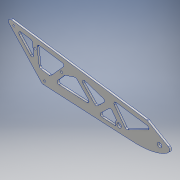
# Autodesk Inventor part: bracket1
Saved by Autodesk Inventor 2018.2 (Build 222227000, 227)
## iProperties
Created: 2018-03-05
Part Number: bracket1
Material: アルミニウム 6061
Document SubType Name: Modeling
Designer: ku_sk
Density: 2.7 g/cm^3
Appearance: アルミニウム - フラット
Mass: 423.846 g
Surface Area: 682.947 cm^2
Volume: 156.98 cm^3
Author: ku_sk
Autodesk Inventor part; units mm, degrees
ref_plane "YZ Plane" through (0, 0, 0) normal (1, 0, 0) x (0, 1, 0)
ref_plane "XZ Plane" through (0, 0, 0) normal (0, 1, 0) x (-1, 0, 0)
ref_plane "XY Plane" through (0, 0, 0) normal (0, 0, 1) x (1, 0, 0)
sketch "スケッチ2" plane through (0, 0, 0) normal (0, 1, 0) x (-1, 0, 0)
  arc A0 (320.7468, 34.8983) -> (392.1215, 71.6787) centre (243.1623, 273.099) ccw projected
  arc A1 (310.5095, 31.8959) -> (320.7468, 34.8983) centre (264.9264, 206.2785) ccw projected
  arc A2 (290.9118, 29.5172) -> (310.5095, 31.8959) centre (291.9468, 102.9093) ccw projected
  arc A3 (278.6891, 31.4878) -> (290.9118, 29.5172) centre (291.5128, 72.1352) ccw projected
  arc A4 (274.9831, 33.389) -> (278.6891, 31.4878) centre (282.4278, 43.3382) ccw projected
  arc A5 (275.4733, 39.2078) -> (274.9831, 33.389) centre (277.0456, 36.1453) ccw projected
  arc A6 (283.1253, 42.3274) -> (275.4733, 39.2078) centre (297.1464, -3.0086) ccw projected
  arc A7 (310.1184, 49.282) -> (283.1253, 42.3274) centre (369.3413, -236.446) ccw projected
  arc A8 (310.1184, 49.282) -> (326.9533, 52.7997) centre (-771.7798, 5269.0252) ccw projected
  arc A9 (326.9533, 52.7997) -> (357.98, 60.8795) centre (256.8539, 385.5961) ccw projected
  arc A10 (357.98, 60.8795) -> (391.1188, 73.3957) centre (268.9975, 346.6028) ccw projected
  arc A11 (392.1215, 71.6787) -> (391.1188, 73.3957) centre (391.5269, 72.4828) ccw projected
  circle A12 centre (287.1934, 37.1564) radius 3 projected
  circle A13 centre (359.7933, 56.2153) radius 3 projected
  arc A14 (100.5026, -29.4375) -> (303.8176, 17.6729) centre (68.6386, 570.3585) ccw projected
  arc A15 (74.9408, -30.0377) -> (100.5026, -29.4375) centre (77.5861, 401.9345) ccw projected
  arc A16 (28.1912, -23.4013) -> (74.9408, -30.0377) centre (76.0159, 145.5175) ccw projected
  arc A17 (1.2395, -11.312) -> (28.1912, -23.4013) centre (55.8939, 74.446) ccw projected
  arc A18 (-6.0217, -4.7376) -> (1.2395, -11.312) centre (16.9451, 13.3315) ccw projected
  arc A19 (-1.6159, 7.4897) -> (-6.0217, -4.7376) centre (0, 0) ccw projected
  arc A20 (17.9572, 9.9554) -> (-1.6159, 7.4897) centre (22.277, -103.2534) ccw projected
  arc A21 (84.7958, 9.311) -> (17.9572, 9.9554) centre (44.6377, -689.2581) ccw projected
  arc A22 (84.7958, 9.311) -> (126.0099, 7.0084) centre (819.0754, 12782.4716) ccw projected
  arc A23 (126.0099, 7.0084) -> (203.0122, 6.466) centre (170.258, 822.6468) ccw projected
  arc A24 (203.0122, 6.466) -> (303.8176, 17.6729) centre (174.1884, 724.7085) ccw projected
  circle A25 centre (20.0666, -1.5588) radius 5 projected
  circle A26 centre (130.4331, -10.1322) radius 5 projected
  line L0 (100.5026, -29.4375) -> (340.2835, -16.6992)
  line L1 (-3.831, 6.6355) -> (54.1787, 40.1274)
  line L2 (1137.2465, 0) -> (-1089.9509, 0) projected
  line L3 (54.1787, 40.1274) -> (443.8225, 95.0028)
  line L4 (340.2835, -16.6992) -> (443.8225, 95.0028)
  point P0 (0, 0)
  point P1 (371.2778, 57.8193)
  dimension "d7" = 30
  constraints: 8 end point, 2 point on circle, 2 tangent
  measures "d7" angle of L2 L1
extrude "押し出し3" add sketch "スケッチ2" along normal blind 5 contours A1 A2 A3 A4 A5 A6 A7 A8 A9 A10 A11 A0 | A15 A16 A17 A18 A19 L2 A25 A14 | A14 L2 L4 L0 | L2 A25 A19 A20 A21 A22 A23 A24 A14 | A14 A24 A23 A22 A21 A20 A19 L1 L3 L4 L2
fillet "フィレット2" radius 6 2 edges at (-54.1787, 2.5, 40.1274) (-340.2835, 2.5, -16.6992)
fillet "フィレット2" radius 7 1 edges at (-443.8225, 2.5, 95.0028)
sketch "スケッチ4" plane through (0, 5, 0) normal (0, 1, 0) x (1, 0, 0)
  circle A0 centre (-333.5539, 7.0426) radius 2.5
  line L0 (-53.1694, -39.5447) -> (3.831, -6.6355) projected
  line L1 (-443.8225, -95.0028) -> (-55.3327, -40.2899) projected
  line L2 (-100.5026, 29.4375) -> (-337.8548, 16.8282) projected
  line L3 (-341.9369, 14.9154) -> (-443.8225, -95.0028) projected
  circle A1 centre (-417.3739, -81.1793) radius 2.5
  point P0 (0, 0)
  dimension "d21" = 5
  dimension "d22" = 10
  dimension "d23" = 11.5
  dimension "d77" = 10
  dimension "d78" = 10
  dimension "d79" = 5
  constraints: 2 centre point
  measures "d21" diameter of A0
  measures "d22" distance from line of L2 A0.centre
  measures "d23" distance from line of L3 A0.centre
  measures "d77" distance from line of A1.centre L1
  measures "d78" distance from line of L3 A1.centre
  measures "d79" diameter of A1
sketch "スケッチ6" plane through (0, 0, 0) normal (0, -1, 0) x (1, 0, 0)
  circle A0 centre (-20.0666, -1.5588) radius 6
  circle A1 centre (-20.0666, -1.5588) radius 5 projected
  circle A2 centre (-130.4331, -10.1322) radius 6
  circle A3 centre (-130.4331, -10.1322) radius 5 projected
  point P0 (0, 0)
  dimension "d29" = 12
  dimension "d30" = 12
  constraints: 2 centre point, 2 concentric
  measures "d29" diameter of A0
  measures "d30" diameter of A2
extrude "押し出し7" cut sketch "スケッチ6" against normal through all
extrude "押し出し9" cut sketch "スケッチ4" against normal through all
sketch "スケッチ7" plane through (0, 0, 0) normal (0, -1, 0) x (1, 0, 0)
  line L0 (-412.0842, 78.4146) -> (-367.524, 72.1389)
  line L1 (-367.524, 72.1389) -> (-360.7767, 23.062)
  line L2 (-360.7767, 23.062) -> (-412.0842, 78.4146)
  line L3 (-424.3323, 92.2579) -> (-55.3327, 40.2899) projected
  line L4 (-341.9369, -14.9154) -> (-430.4423, 80.5677) projected
  line L5 (-355.1719, 70.3993) -> (-347.8097, 16.8493)
  line L6 (-347.8097, 16.8493) -> (-317.9372, 12.6422)
  line L7 (-317.9372, 12.6422) -> (-275.9537, 59.2426)
  line L8 (-275.9537, 59.2426) -> (-355.1719, 70.3993)
  line L9 (-304.865, 4.742) -> (-205.0058, -0.563)
  line L10 (-205.0058, -0.563) -> (-248.1507, 44.1788)
  line L11 (-248.1507, 44.1788) -> (-278.0912, 34.4601)
  line L12 (-278.0912, 34.4601) -> (-304.865, 4.742)
  line L13 (-100.5026, -29.4375) -> (-337.8548, -16.8282) projected
  line L14 (-193.1155, 2.9534) -> (-242.9077, 54.5886)
  line L15 (-242.9077, 54.5886) -> (-165.6606, 29.4284)
  line L16 (-165.6606, 29.4284) -> (-193.1155, 2.9534)
  line L17 (-150.8906, 41.6294) -> (-111.4803, -10.7012)
  line L18 (-111.4803, -10.7012) -> (-37.0144, 25.5916)
  line L19 (-37.0144, 25.5916) -> (-150.8906, 41.6294)
  line L20 (-153.5684, 20.2509) -> (-188.5225, -13.4556)
  line L21 (-188.5225, -13.4556) -> (-125.6693, -16.7947)
  line L22 (-125.6693, -16.7947) -> (-153.5684, 20.2509)
  point P0 (0, 0)
  dimension "d82" = 12
  dimension "d83" = 12
  dimension "d84" = 35
  dimension "d85" = 12
  dimension "d86" = 45
  dimension "d87" = 56
  dimension "d88" = 52
  dimension "d89" = 80
  dimension "d90" = 15
  dimension "d91" = 30
  dimension "d92" = 40
  dimension "d93" = 100
  dimension "d94" = 43
  dimension "d95" = 6
  dimension "d96" = 28
  dimension "d97" = 11
  dimension "d99" = 90
  dimension "d100" = 12
  dimension "d101" = 45
  dimension "d102" = 34
  dimension "d103" = 115
  dimension "d104" = 45
  dimension "d108" = 12
  dimension "d109" = 15
  dimension "d110" = 15
  constraints: 40 end point, 11 parallel, 2 point on line, 1 collinear
  measures "d82" distance between parallel lines of L0 L3
  measures "d83" distance between parallel lines of L4 L2
  measures "d84" angle of L2 L1
  measures "d85" distance between parallel lines of L5 L1
  measures "d86" distance of L0.start L0.end
  measures "d87" angle of L7 L8
  measures "d88" distance between parallel lines of L8 L6
  measures "d89" distance of L7.end L5.start
  measures "d90" distance between parallel lines of L12 L7
  measures "d91" angle of L12 L11
  measures "d92" distance of L11.end L9.start
  measures "d93" distance of L9.start L9.end
  measures "d94" angle of L9 L10
  measures "d95" distance from line of L9.start L6
  measures "d96" angle of L14 L15
  measures "d97" distance between parallel lines of L10 L14
  measures "d99" angle of L14 L16
  measures "d100" distance between parallel lines of L19 L3
  measures "d101" angle of L17 L19
  measures "d102" angle of L18 L19
  measures "d103" distance of L18.end L17.start
  measures "d104" distance of point (0, 0) L18.end
  measures "d108" distance between parallel lines of L9 L21
  measures "d109" distance between parallel lines of L17 L22
  measures "d110" distance between parallel lines of L16 L20
extrude "押し出し10" cut sketch "スケッチ7" against normal through all
fillet "フィレット3" radius 5 20 edges at (-412.0842, 2.5, 78.4146) (-355.1719, 2.5, 70.3993) (-278.0912, 2.5, 34.4601) (-242.9077, 2.5, 54.5886) (-150.8906, 2.5, 41.6294) (-111.4803, 2.5, -10.7012) (-193.1155, 2.5, 2.9534) (-317.9372, 2.5, 12.6422) (-360.7767, 2.5, 23.062) (-367.524, 2.5, 72.1389) (-275.9537, 2.5, 59.2426) (-37.0144, 2.5, 25.5916) (-165.6606, 2.5, 29.4284) (-248.1507, 2.5, 44.1788) (-153.5684, 2.5, 20.2509) (-188.5225, 2.5, -13.4556) (-304.865, 2.5, 4.742) (-347.8097, 2.5, 16.8493) (-205.0058, 2.5, -0.563) (-125.6693, 2.5, -16.7947)
sketch "スケッチ8" plane through (0, 0, 0) normal (0, -1, 0) x (1, 0, 0)
  circle A0 centre (-130.4331, -10.1322) radius 11
  circle A1 centre (-130.4331, -10.1322) radius 6
  arc A2 (-126.9876, -15.0443) -> (-134.2025, -5.464) centre (-130.4331, -10.1322) ccw projected
  point P0 (0, 0)
  dimension "d111" = 12
  dimension "d112" = 5
  constraints: 2 centre point, 1 coincident, 1 concentric
  measures "d111" diameter of A1
  measures "d112" radial gap between concentric circles of A1 A0
extrude "押し出し11" add sketch "スケッチ8" against normal blind 5
